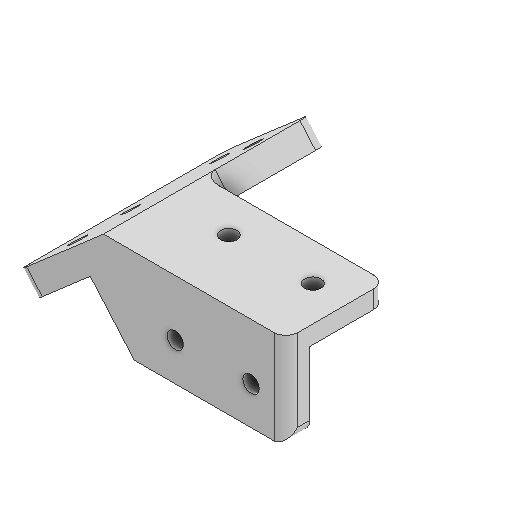
# Autodesk Inventor part: frontUndercarriageBracketFlipped
Saved by Autodesk Inventor 2025 (Build 290162000, 162)
## iProperties
Created: 2024-12-12
Part Number: frontUndercarriageBracketFlipped
Material: Generic
Document SubType Name: Modeling
Designer: derm
Density: 1 g/cm^3
Appearance: Default
Author: derm
Autodesk Inventor part; units mm, degrees
ref_plane "YZ Plane" through (0, 0, 0) normal (1, 0, 0) x (0, 1, 0)
ref_plane "XZ Plane" through (0, 0, 0) normal (0, 1, 0) x (-1, 0, 0)
ref_plane "XY Plane" through (0, 0, 0) normal (0, 0, 1) x (1, 0, 0)
sketch "Sketch1" plane through (0, 0, 0) normal (0, 0, 1) x (1, 0, 0)
  line L0 (0, 0) -> (50.8, 0)
  line L1 (50.8, 0) -> (50.8, 25.4)
  line L2 (50.8, 25.4) -> (0, 25.4)
  line L3 (0, 25.4) -> (0, 0)
  circle A0 centre (13.7086, 12.7) radius 2.75
  circle A1 centre (39.1086, 12.7) radius 2.75
  point P0 (50.8, 12.7)
  dimension "d0" = 25.4
  dimension "d1" = 50.8
  dimension "d2" = 5.5
  dimension "d3" = 5.5
  dimension "d4" = 25.4
  constraints: 8 end point, 2 centre point, 2 parallel, 1 horizontal, 1 midpoint, 1 perpendicular
  measures "d0" distance between parallel lines of L0 L2
  measures "d1" distance from line of point (50.8, 12.7) L3
  measures "d2" diameter of A0
  measures "d3" diameter of A1
  measures "d4" distance of A1.centre A0.centre
extrude "Extrusion1" add sketch "Sketch1" along normal blind 8
sketch "Sketch2" plane through (0, 0, 0) normal (0, 0, -1) x (-1, 0, 0)
  line L0 (-50.8, 0) -> (-50.8, 25.4) projected
  line L1 (0, 0) -> (-50.8, 0) projected
  line L2 (0, 25.4) -> (0, 0) projected
  line L3 (-50.8, 25.4) -> (0, 25.4) projected
  circle A0 centre (-13.7086, 12.7) radius 2.75 projected
  circle A1 centre (-39.1086, 12.7) radius 2.75 projected
  line L4 (8.7026, 22.2526) -> (-37.7738, 62.6539) projected
  line L5 (0, 25.4) -> (5.082, 25.4)
  line L6 (0, 0) -> (14.7638, 16.9838)
  line L7 (14.7638, 16.9838) -> (5.082, 25.4)
  constraints: 6 end point, 2 point on line, 1 collinear, 1 horizontal, 1 perpendicular
extrude "Extrusion2" add sketch "Sketch2" against normal blind 33.4 contours L2 L5 L4 L7 L6
sketch "Sketch3" plane through (-14.7638, 16.9838, 33.4) normal (-0.656059, 0.7547096, 0) x (0.7547096, 0.656059, 0)
  line L0 (-25.28, -11.14) -> (-25.28, 242.86)
  line L1 (519.5133, -36.42) -> (-90.0867, -36.42)
  line L2 (0, 33.4) -> (12.8285, 33.4)
  line L3 (0, 33.4) -> (0, 0)
  line L4 (12.8285, 0) -> (0, 0)
  line L5 (12.8285, 33.4) -> (12.8285, 0)
  line L6 (12.8285, 33.4) -> (-25.28, 33.4)
  line L7 (-25.28, 33.4) -> (-25.28, -36.42)
  line L8 (-25.28, -36.42) -> (12.8285, -36.42)
  line L9 (12.8285, -36.42) -> (12.8285, 33.4)
  line L10 (-9.4488, -11.14) -> (-9.4488, 242.86)
  line L11 (-15.9512, -11.14) -> (-15.9512, 242.86)
  line L12 (519.5133, -20.5888) -> (-90.0867, -20.5888)
  line L13 (519.5133, -27.0912) -> (-90.0867, -27.0912)
  circle A0 centre (-12.6415, 22.815) radius 2.75
  circle A1 centre (-12.6415, 5.0274) radius 2.75
  circle A2 centre (-12.1988, -24.4757) radius 2.75
  circle A3 centre (2.7133, -24.4757) radius 2.75
  point P0 (0, 33.4)
  point P1 (12.8285, -36.42)
  point P2 (12.8285, 0)
extrude "Extrusion3" add sketch "Sketch3" along normal blind 8 contours L0 L6 L3 L4 L9 L12 L7 | L12 L9 L13 A3 A2 L7 | L13 A2 A3 L9 L1 L7 | L4 L3 L2 L5
sketch "Sketch4" plane through (0, 0, 0) normal (0, 0, -1) x (-1, 0, 0)
  line L0 (-50.8, 0) -> (-50.8, 25.4) projected
  line L1 (0, 0) -> (-50.8, 0) projected
  line L2 (0, 0) -> (14.7638, 16.9838) projected
  line L3 (14.7638, 16.9838) -> (33.8428, 0.3986) projected
  line L4 (33.8428, 0.3986) -> (39.0913, 6.4363) projected
  line L5 (10.3305, 31.4377) -> (39.0913, 6.4363) projected
  line L6 (5.082, 25.4) -> (10.3305, 31.4377) projected
  line L7 (-50.8, 25.4) -> (5.082, 25.4) projected
  circle A0 centre (-13.7086, 12.7) radius 2.75 projected
  circle A1 centre (-39.1086, 12.7) radius 2.75 projected
  line L8 (-50.8, 25.4) -> (-50.8, 31.4377)
  line L9 (-50.8, 31.4377) -> (10.3305, 31.4377)
  constraints: 4 end point, 1 vertical
extrude "Extrusion4" add sketch "Sketch4" against normal up to surface (33.4 mm away) contours L8 L9 L6 L7
sketch "Sketch5" plane through (-10.3305, 31.4377, 0) normal (0, 1, 0) x (1, 0, 0)
  line L0 (61.1305, -33.4) -> (0, -33.4) projected
  line L1 (61.1305, 0) -> (61.1305, -33.4) projected
  line L2 (0, 0) -> (61.1305, 0) projected
  line L3 (0, -33.4) -> (0, 0) projected
  line L4 (61.1305, -8) -> (10.3305, -8) projected
  line L5 (52.1891, 0) -> (46.6891, 0) projected
  line L6 (26.7891, 0) -> (21.2891, 0) projected
  circle A0 centre (49.4391, -20.7) radius 2.75
  circle A1 centre (21.2891, -20.7) radius 2.75
  point P0 (10.3305, 0)
  constraints: 2 centre point
extrude "Extrusion5" cut sketch "Sketch5" against normal through all contours A0 | A1
fillet "Fillet1" radius 2 1 edges at (0, 0, 20.7)
fillet "Fillet2" radius 4 7 edges at (-36.467, 3.4174, 0) (-36.467, 3.4174, 69.82) (-7.7062, 28.4188, 69.82) (-7.7062, 28.4188, 33.4) (50.8, 28.4188, 33.4) (50.8, 0, 4) (50.8, 15.7188, 0)
mirror "Mirror1" about plane through (25.4, 12.7, 0) normal (0, 0, -1) remove original yes
body "Solid1"
